Autodesk Fusion 360 part; units mm, degrees
(part 3 of 6)
  spline S740 degree 3 poles (-68.6412, -18.0684) (-68.8412, -19.3768) (-68.5019, -20.6874) (-67.7379, -21.7563) knots 0 0 0 0 1 1 1 1
  spline S741 degree 3 poles (-67.7379, -21.7563) (-67.4869, -22.0922) (-67.1872, -22.3895) (-66.7921, -22.5521) knots 0 0 0 0 1 1 1 1
  spline S742 degree 3 poles (-66.7921, -22.5521) (-66.7066, -22.5523) (-66.7066, -22.5523) (-66.6238, -22.5405) knots 0 0 0 0 1 1 1 1
  spline S743 degree 3 poles (-66.6238, -22.5405) (-66.5712, -22.5389) (-66.5187, -22.5373) (-66.4646, -22.5356) knots 0 0 0 0 1 1 1 1
  spline S744 degree 3 poles (-66.4646, -22.5356) (-66.4043, -22.5997) (-66.4043, -22.5997) (-66.3562, -22.6818) knots 0 0 0 0 1 1 1 1
  spline S745 degree 3 poles (-66.3562, -22.6818) (-66.0629, -23.057) (-65.7293, -23.2124) (-65.2682, -23.3032) knots 0 0 0 0 1 1 1 1
  spline S746 degree 3 poles (-65.2682, -23.3032) (-64.8355, -23.3775) (-64.8355, -23.3775) (-64.5079, -23.6467) knots 0 0 0 0 1 1 1 1
  spline S747 degree 3 poles (-64.5079, -23.6467) (-64.3934, -23.7401) (-64.3934, -23.7401) (-64.303, -23.7316) knots 0 0 0 0 1 1 1 1
  spline S748 degree 3 poles (-64.303, -23.7316) (-64.2502, -23.719) (-64.2502, -23.719) (-64.1964, -23.706) knots 0 0 0 0 1 1 1 1
  spline S749 degree 3 poles (-64.1964, -23.706) (-63.9469, -23.6555) (-63.7172, -23.6642) (-63.4643, -23.6796) knots 0 0 0 0 1 1 1 1
  spline S750 degree 3 poles (-63.4643, -23.6796) (-62.4889, -23.724) (-62.4889, -23.724) (-62.1287, -23.4647) knots 0 0 0 0 1 1 1 1
  spline S751 degree 3 poles (-62.1287, -23.4647) (-62.0488, -23.3538) (-61.9871, -23.2352) (-61.9247, -23.1138) knots 0 0 0 0 1 1 1 1
  spline S752 degree 3 poles (-61.9247, -23.1138) (-61.8889, -23.0471) (-61.8532, -22.9804) (-61.8173, -22.9138) knots 0 0 0 0 1 1 1 1
  spline S753 degree 3 poles (-61.8173, -22.9138) (-61.7921, -22.8662) (-61.7921, -22.8662) (-61.7664, -22.8176) knots 0 0 0 0 1 1 1 1
  spline S754 degree 3 poles (-61.7664, -22.8176) (-61.5666, -22.4407) (-61.3314, -22.1103) (-60.9949, -21.8423) knots 0 0 0 0 1 1 1 1
  spline S755 degree 3 poles (-60.9949, -21.8423) (-60.8309, -21.6988) (-60.7879, -21.5385) (-60.7711, -21.3252) knots 0 0 0 0 1 1 1 1
  spline S756 degree 3 poles (-60.7711, -21.3252) (-60.7791, -21.0767) (-60.8479, -20.9431) (-60.9972, -20.7455) knots 0 0 0 0 1 1 1 1
  spline S757 degree 3 poles (-60.9972, -20.7455) (-61.0269, -20.5521) (-60.9721, -20.3858) (-60.9221, -20.2004) knots 0 0 0 0 1 1 1 1
  spline S758 degree 3 poles (-60.9221, -20.2004) (-60.8997, -20.0941) (-60.9058, -20.0126) (-60.9382, -19.9089) knots 0 0 0 0 1 1 1 1
  spline S759 degree 3 poles (-60.9382, -19.9089) (-60.9049, -19.8925) (-60.8717, -19.8761) (-60.8374, -19.8592) knots 0 0 0 0 1 1 1 1
  spline S760 degree 3 poles (-60.8374, -19.8592) (-60.5508, -19.6929) (-60.3089, -19.433) (-60.2049, -19.1155) knots 0 0 0 0 1 1 1 1
  spline S761 degree 3 poles (-60.2049, -19.1155) (-60.1104, -18.7393) (-60.169, -18.4062) (-60.3535, -18.0709) knots 0 0 0 0 1 1 1 1
  spline S762 degree 3 poles (-60.3535, -18.0709) (-60.3718, -17.8493) (-60.3514, -17.638) (-60.3266, -17.4182) knots 0 0 0 0 1 1 1 1
  spline S763 degree 3 poles (-60.3266, -17.4182) (-60.2811, -16.9783) (-60.2704, -16.5662) (-60.3651, -16.1315) knots 0 0 0 0 1 1 1 1
  spline S764 degree 3 poles (-60.3651, -16.1315) (-60.3404, -16.1338) (-60.3158, -16.1361) (-60.2904, -16.1385) knots 0 0 0 0 1 1 1 1
  spline S765 degree 3 poles (-60.2904, -16.1385) (-60.0658, -16.1502) (-59.8801, -16.0893) (-59.6783, -16.0001) knots 0 0 0 0 1 1 1 1
  spline S766 degree 3 poles (-59.6783, -16.0001) (-59.3356, -15.8722) (-59.0125, -15.9703) (-58.6693, -16.0524) knots 0 0 0 0 1 1 1 1
  spline S767 degree 3 poles (-58.6693, -16.0524) (-56.6827, -16.5272) (-54.5948, -16.1567) (-52.6142, -15.7994) knots 0 0 0 0 1 1 1 1
  spline S768 degree 3 poles (-52.6142, -15.7994) (-52.425, -15.7652) (-52.2358, -15.7315) (-52.0466, -15.6978) knots 0 0 0 0 1 1 1 1
  spline S769 degree 3 poles (-52.0466, -15.6978) (-51.5093, -15.6021) (-50.9721, -15.5059) (-50.4349, -15.4093) knots 0 0 0 0 1 1 1 1
  spline S770 degree 3 poles (-50.4349, -15.4093) (-50.1364, -15.3556) (-49.8377, -15.3022) (-49.539, -15.2492) knots 0 0 0 0 1 1 1 1
  spline S771 degree 3 poles (-49.539, -15.2492) (-49.3825, -15.2214) (-49.2259, -15.1934) (-49.0695, -15.165) knots 0 0 0 0 1 1 1 1
  spline S772 degree 3 poles (-49.0695, -15.165) (-47.9373, -14.9598) (-46.7937, -14.7812) (-45.6425, -14.736) knots 0 0 0 0 1 1 1 1
  spline S773 degree 3 poles (-45.6425, -14.736) (-45.5861, -14.7334) (-45.5298, -14.7307) (-45.4735, -14.7279) knots 0 0 0 0 1 1 1 1
  spline S774 degree 3 poles (-45.4735, -14.7279) (-45.2474, -14.7174) (-45.0218, -14.7091) (-44.7954, -14.708) knots 0 0 0 0 1 1 1 1
  spline S775 degree 3 poles (-44.7954, -14.708) (-44.7994, -14.7532) (-44.8034, -14.7983) (-44.8075, -14.8449) knots 0 0 0 0 1 1 1 1
  spline S776 degree 3 poles (-44.8075, -14.8449) (-44.8816, -15.7919) (-44.8816, -15.7919) (-44.6213, -16.1643) knots 0 0 0 0 1 1 1 1
  spline S777 degree 3 poles (-44.6213, -16.1643) (-44.5265, -16.2347) (-44.4252, -16.2864) (-44.3195, -16.3383) knots 0 0 0 0 1 1 1 1
  spline S778 degree 3 poles (-44.3195, -16.3383) (-44.2905, -16.353) (-44.2615, -16.3677) (-44.2317, -16.3828) knots 0 0 0 0 1 1 1 1
  spline S779 degree 3 poles (-44.2317, -16.3828) (-44.1742, -16.4117) (-44.1167, -16.4403) (-44.0589, -16.4685) knots 0 0 0 0 1 1 1 1
  spline S780 degree 3 poles (-44.0589, -16.4685) (-43.9984, -16.4984) (-43.9388, -16.53) (-43.8796, -16.5622) knots 0 0 0 0 1 1 1 1
  spline S781 degree 3 poles (-43.8796, -16.5622) (-43.2204, -16.8977) (-42.2928, -16.9139) (-41.572, -16.8246) knots 0 0 0 0 1 1 1 1
  spline S782 degree 3 poles (-41.572, -16.8246) (-41.5398, -16.823) (-41.5077, -16.8213) (-41.4745, -16.8197) knots 0 0 0 0 1 1 1 1
  spline S783 degree 3 poles (-41.4745, -16.8197) (-41.3362, -16.8073) (-41.2458, -16.7972) (-41.1479, -16.694) knots 0 0 0 0 1 1 1 1
  spline S784 degree 3 poles (-41.1479, -16.694) (-40.9639, -16.4028) (-40.9726, -16.1477) (-41.0367, -15.8177) knots 0 0 0 0 1 1 1 1
  spline S785 degree 3 poles (-41.0367, -15.8177) (-41.094, -15.6049) (-41.2091, -15.4396) (-41.3857, -15.3047) knots 0 0 0 0 1 1 1 1
  spline S786 degree 3 poles (-41.3857, -15.3047) (-41.4121, -15.3093) (-41.4385, -15.314) (-41.4658, -15.3188) knots 0 0 0 0 1 1 1 1
  spline S787 degree 3 poles (-41.4658, -15.3188) (-41.4806, -15.2976) (-41.4954, -15.2763) (-41.5107, -15.2544) knots 0 0 0 0 1 1 1 1
  spline S788 degree 3 poles (-41.5107, -15.2544) (-41.5751, -15.1714) (-41.6453, -15.1045) (-41.7226, -15.0336) knots 0 0 0 0 1 1 1 1
  spline S789 degree 3 poles (-41.7226, -15.0336) (-41.6474, -15.0014) (-41.5722, -14.9692) (-41.497, -14.937) knots 0 0 0 0 1 1 1 1
  spline S790 degree 3 poles (-41.497, -14.937) (-41.4514, -14.9175) (-41.4058, -14.8979) (-41.3588, -14.8777) knots 0 0 0 0 1 1 1 1
  spline S791 degree 3 poles (-41.3588, -14.8777) (-41.2453, -14.8308) (-41.1322, -14.7907) (-41.0159, -14.7515) knots 0 0 0 0 1 1 1 1
  spline S792 degree 3 poles (-41.0159, -14.7515) (-40.6691, -14.6161) (-40.4632, -14.2783) (-40.3015, -13.9569) knots 0 0 0 0 1 1 1 1
  spline S793 degree 3 poles (-40.3015, -13.9569) (-40.2178, -13.7291) (-40.1926, -13.5214) (-40.2142, -13.2806) knots 0 0 0 0 1 1 1 1
  spline S794 degree 3 poles (-40.2142, -13.2806) (-40.105, -13.2803) (-40.0232, -13.2817) (-39.9196, -13.3113) knots 0 0 0 0 1 1 1 1
  spline S795 degree 3 poles (-39.9196, -13.3113) (-39.828, -13.4095) (-39.828, -13.4095) (-39.7728, -13.4871) knots 0 0 0 0 1 1 1 1
  spline S796 degree 3 poles (-39.7728, -13.4871) (-39.1827, -14.2043) (-38.1238, -14.3933) (-37.2636, -14.5675) knots 0 0 0 0 1 1 1 1
  spline S797 degree 3 poles (-37.2636, -14.5675) (-37.1583, -14.5891) (-37.053, -14.6108) (-36.9477, -14.6327) knots 0 0 0 0 1 1 1 1
  spline S798 degree 3 poles (-36.9477, -14.6327) (-36.8831, -14.6461) (-36.8183, -14.6593) (-36.7536, -14.6724) knots 0 0 0 0 1 1 1 1
  spline S799 degree 3 poles (-36.7536, -14.6724) (-36.5691, -14.7103) (-36.3908, -14.7577) (-36.2115, -14.8155) knots 0 0 0 0 1 1 1 1
  spline S800 degree 3 poles (-36.2115, -14.8155) (-36.14, -14.8341) (-36.14, -14.8341) (-36.0599, -14.82) knots 0 0 0 0 1 1 1 1
  spline S801 degree 3 poles (-36.0599, -14.82) (-36.0685, -14.8488) (-36.077, -14.8775) (-36.0858, -14.9072) knots 0 0 0 0 1 1 1 1
  spline S802 degree 3 poles (-36.0858, -14.9072) (-36.1556, -14.9418) (-36.1556, -14.9418) (-36.244, -14.9684) knots 0 0 0 0 1 1 1 1
  spline S803 degree 3 poles (-36.244, -14.9684) (-36.2782, -14.9796) (-36.3123, -14.9909) (-36.3475, -15.0025) knots 0 0 0 0 1 1 1 1
  spline S804 degree 3 poles (-36.3475, -15.0025) (-36.385, -15.0145) (-36.4225, -15.0265) (-36.4612, -15.0389) knots 0 0 0 0 1 1 1 1
  spline S805 degree 3 poles (-36.4612, -15.0389) (-36.4999, -15.0515) (-36.5387, -15.0642) (-36.5786, -15.0773) knots 0 0 0 0 1 1 1 1
  spline S806 degree 3 poles (-36.5786, -15.0773) (-36.6619, -15.1045) (-36.7452, -15.1316) (-36.8286, -15.1585) knots 0 0 0 0 1 1 1 1
  spline S807 degree 3 poles (-36.8286, -15.1585) (-36.958, -15.2003) (-37.0873, -15.2425) (-37.2165, -15.2849) knots 0 0 0 0 1 1 1 1
  spline S808 degree 3 poles (-37.2165, -15.2849) (-37.5564, -15.3961) (-37.8965, -15.5064) (-38.2368, -15.6164) knots 0 0 0 0 1 1 1 1
  spline S809 degree 3 poles (-38.2368, -15.6164) (-38.3584, -15.6559) (-38.4799, -15.6957) (-38.6015, -15.7354) knots 0 0 0 0 1 1 1 1
  spline S810 degree 3 poles (-38.6015, -15.7354) (-38.6442, -15.749) (-38.6869, -15.7626) (-38.7309, -15.7766) knots 0 0 0 0 1 1 1 1
  spline S811 degree 3 poles (-38.7309, -15.7766) (-38.7688, -15.789) (-38.8066, -15.8014) (-38.8456, -15.8141) knots 0 0 0 0 1 1 1 1
  spline S812 degree 3 poles (-38.8456, -15.8141) (-38.8777, -15.8244) (-38.9098, -15.8347) (-38.9428, -15.8454) knots 0 0 0 0 1 1 1 1
  spline S813 degree 3 poles (-38.9428, -15.8454) (-38.9659, -15.856) (-38.989, -15.8667) (-39.0127, -15.8776) knots 0 0 0 0 1 1 1 1
  spline S814 degree 3 poles (-39.0127, -15.8776) (-39.064, -16.0501) (-39.0117, -16.2422) (-38.9897, -16.4183) knots 0 0 0 0 1 1 1 1
  spline S815 degree 3 poles (-38.9897, -16.4183) (-38.9829, -16.4809) (-38.9829, -16.4809) (-38.976, -16.5447) knots 0 0 0 0 1 1 1 1
  spline S816 degree 3 poles (-38.976, -16.5447) (-38.9451, -16.7912) (-38.9094, -16.9616) (-38.7466, -17.1525) knots 0 0 0 0 1 1 1 1
  spline S817 degree 3 poles (-38.7466, -17.1525) (-38.5182, -17.2701) (-38.3218, -17.2898) (-38.0703, -17.2398) knots 0 0 0 0 1 1 1 1
  spline S818 degree 3 poles (-38.0703, -17.2398) (-37.993, -17.2137) (-37.9161, -17.1863) (-37.8395, -17.1578) knots 0 0 0 0 1 1 1 1
  spline S819 degree 3 poles (-37.8395, -17.1578) (-37.0677, -16.8843) (-36.2352, -16.9908) (-35.4358, -17.0521) knots 0 0 0 0 1 1 1 1
  spline S820 degree 3 poles (-35.4358, -17.0521) (-34.7031, -17.1078) (-34.0053, -17.132) (-33.2842, -16.9742) knots 0 0 0 0 1 1 1 1
  spline S821 degree 3 poles (-33.2842, -16.9742) (-33.276, -17.0018) (-33.2678, -17.0295) (-33.2593, -17.0579) knots 0 0 0 0 1 1 1 1
  spline S822 degree 3 poles (-33.2593, -17.0579) (-33.0671, -17.4752) (-32.5518, -17.7504) (-32.1451, -17.9145) knots 0 0 0 0 1 1 1 1
  spline S823 degree 3 poles (-32.1451, -17.9145) (-31.6456, -18.089) (-31.1293, -18.1169) (-30.6051, -18.1128) knots 0 0 0 0 1 1 1 1
  spline S824 degree 3 poles (-30.6051, -18.1128) (-30.5551, -18.1131) (-30.5052, -18.1134) (-30.4537, -18.1137) knots 0 0 0 0 1 1 1 1
  spline S825 degree 3 poles (-30.4537, -18.1137) (-30.2637, -18.0993) (-30.1747, -18.031) (-30.0183, -17.9267) knots 0 0 0 0 1 1 1 1
  spline S826 degree 3 poles (-30.0183, -17.9267) (-29.9953, -17.9746) (-29.9724, -18.0225) (-29.9488, -18.0719) knots 0 0 0 0 1 1 1 1
  spline S827 degree 3 poles (-29.9488, -18.0719) (-29.6863, -18.5524) (-29.2614, -18.9058) (-28.739, -19.0617) knots 0 0 0 0 1 1 1 1
  spline S828 degree 3 poles (-28.739, -19.0617) (-28.3779, -19.1626) (-28.0211, -19.2161) (-27.668, -19.0613) knots 0 0 0 0 1 1 1 1
  spline S829 degree 3 poles (-27.668, -19.0613) (-27.5114, -18.9684) (-27.4277, -18.8659) (-27.3626, -18.6976) knots 0 0 0 0 1 1 1 1
  spline S830 degree 3 poles (-27.3626, -18.6976) (-27.3559, -18.5596) (-27.3559, -18.5596) (-27.3649, -18.4502) knots 0 0 0 0 1 1 1 1
  spline S831 degree 3 poles (-27.3649, -18.4502) (-27.1789, -18.5763) (-27.0065, -18.7141) (-26.8336, -18.8574) knots 0 0 0 0 1 1 1 1
  spline S832 degree 3 poles (-26.8336, -18.8574) (-25.8457, -19.6635) (-24.4693, -20.4549) (-23.14, -20.3902) knots 0 0 0 0 1 1 1 1
  spline S833 degree 3 poles (-23.14, -20.3902) (-22.9866, -20.3473) (-22.9116, -20.291) (-22.8156, -20.1652) knots 0 0 0 0 1 1 1 1
  spline S834 degree 3 poles (-22.8156, -20.1652) (-22.7953, -20.139) (-22.7749, -20.1128) (-22.754, -20.0857) knots 0 0 0 0 1 1 1 1
  spline S835 degree 3 poles (-22.754, -20.0857) (-22.739, -20.0657) (-22.7241, -20.0457) (-22.7087, -20.025) knots 0 0 0 0 1 1 1 1
  spline S836 degree 3 poles (-22.7087, -20.025) (-22.6443, -20.1421) (-22.5821, -20.2595) (-22.5234, -20.3796) knots 0 0 0 0 1 1 1 1
  spline S837 degree 3 poles (-22.5234, -20.3796) (-21.9291, -21.5595) (-20.6318, -22.2811) (-19.4264, -22.7095) knots 0 0 0 0 1 1 1 1
  spline S838 degree 3 poles (-19.4264, -22.7095) (-18.9788, -22.8304) (-18.5829, -22.8182) (-18.1633, -22.6107) knots 0 0 0 0 1 1 1 1
  spline S839 degree 3 poles (-18.1633, -22.6107) (-18.0483, -22.5271) (-17.9669, -22.4305) (-17.8852, -22.3138) knots 0 0 0 0 1 1 1 1
  spline S840 degree 3 poles (-17.8852, -22.3138) (-17.8567, -22.0715) (-17.9152, -21.8824) (-18.0605, -21.6893) knots 0 0 0 0 1 1 1 1
  spline S841 degree 3 poles (-18.0605, -21.6893) (-18.2688, -21.4713) (-18.5357, -21.3675) (-18.8195, -21.2824) knots 0 0 0 0 1 1 1 1
  spline S842 degree 3 poles (-18.8195, -21.2824) (-18.9043, -21.2593) (-18.9043, -21.2593) (-18.9526, -21.1802) knots 0 0 0 0 1 1 1 1
  spline S843 degree 3 poles (-18.9526, -21.1802) (-18.9261, -21.1665) (-18.8997, -21.1529) (-18.8724, -21.1388) knots 0 0 0 0 1 1 1 1
  spline S844 degree 3 poles (-18.8724, -21.1388) (-18.7401, -21.0464) (-18.6537, -20.9322) (-18.5594, -20.8037) knots 0 0 0 0 1 1 1 1
  spline S845 degree 3 poles (-18.5594, -20.8037) (-18.5331, -20.7686) (-18.5331, -20.7686) (-18.5062, -20.7329) knots 0 0 0 0 1 1 1 1
  spline S846 degree 3 poles (-18.5062, -20.7329) (-18.4236, -20.6226) (-18.3424, -20.5115) (-18.2644, -20.3979) knots 0 0 0 0 1 1 1 1
  spline S847 degree 3 poles (-18.2644, -20.3979) (-18.2324, -20.4233) (-18.2004, -20.4486) (-18.1674, -20.4748) knots 0 0 0 0 1 1 1 1
  spline S848 degree 3 poles (-18.1674, -20.4748) (-17.7298, -20.8181) (-17.2734, -21.1066) (-16.7784, -21.3598) knots 0 0 0 0 1 1 1 1
  spline S849 degree 3 poles (-16.7784, -21.3598) (-16.5763, -21.4634) (-16.3766, -21.5705) (-16.179, -21.6825) knots 0 0 0 0 1 1 1 1
  spline S850 degree 3 poles (-16.179, -21.6825) (-16.1408, -21.7041) (-16.1026, -21.7256) (-16.0633, -21.7478) knots 0 0 0 0 1 1 1 1
  spline S851 degree 3 poles (-16.0633, -21.7478) (-15.8503, -21.8737) (-15.6798, -22.003) (-15.5076, -22.1812) knots 0 0 0 0 1 1 1 1
  spline S852 degree 3 poles (-15.5076, -22.1812) (-15.1305, -22.5482) (-14.4719, -22.7942) (-13.9467, -22.7924) knots 0 0 0 0 1 1 1 1
  spline S853 degree 3 poles (-13.9467, -22.7924) (-13.7622, -22.7691) (-13.6383, -22.6968) (-13.5022, -22.5737) knots 0 0 0 0 1 1 1 1
  spline S854 degree 3 poles (-13.5022, -22.5737) (-13.4682, -22.5272) (-13.4352, -22.4801) (-13.4032, -22.4323) knots 0 0 0 0 1 1 1 1
  spline S855 degree 3 poles (-13.4032, -22.4323) (-13.3735, -22.4075) (-13.3438, -22.3826) (-13.3132, -22.357) knots 0 0 0 0 1 1 1 1
  spline S856 degree 3 poles (-13.3132, -22.357) (-13.1964, -22.2519) (-13.14, -22.1775) (-13.1248, -22.0182) knots 0 0 0 0 1 1 1 1
  spline S857 degree 3 poles (-13.1248, -22.0182) (-13.1272, -21.6444) (-13.2828, -21.3286) (-13.5456, -21.0684) knots 0 0 0 0 1 1 1 1
  spline S858 degree 3 poles (-13.5456, -21.0684) (-13.7172, -20.9144) (-13.8973, -20.7722) (-14.0803, -20.632) knots 0 0 0 0 1 1 1 1
  spline S859 degree 3 poles (-14.0803, -20.632) (-14.5227, -20.289) (-14.9136, -19.9414) (-15.1701, -19.4393) knots 0 0 0 0 1 1 1 1
  spline S860 degree 3 poles (-15.1701, -19.4393) (-15.0261, -19.4638) (-14.8823, -19.4895) (-14.7385, -19.5155) knots 0 0 0 0 1 1 1 1
  spline S861 degree 3 poles (-14.7385, -19.5155) (-14.698, -19.5224) (-14.6574, -19.5293) (-14.6157, -19.5364) knots 0 0 0 0 1 1 1 1
  spline S862 degree 3 poles (-14.6157, -19.5364) (-14.3073, -19.5929) (-14.0901, -19.6827) (-13.8472, -19.885) knots 0 0 0 0 1 1 1 1
  spline S863 degree 3 poles (-13.8472, -19.885) (-13.8189, -19.9083) (-13.7906, -19.9316) (-13.7615, -19.9556) knots 0 0 0 0 1 1 1 1
  spline S864 degree 3 poles (-13.7615, -19.9556) (-13.7279, -19.9836) (-13.6943, -20.0116) (-13.6597, -20.0404) knots 0 0 0 0 1 1 1 1
  spline S865 degree 3 poles (-13.6597, -20.0404) (-11.7063, -21.6601) (-11.7063, -21.6601) (-10.6489, -21.5847) knots 0 0 0 0 1 1 1 1
  spline S866 degree 3 poles (-10.6489, -21.5847) (-10.4516, -21.556) (-10.2712, -21.5209) (-10.1149, -21.3918) knots 0 0 0 0 1 1 1 1
  spline S867 degree 3 poles (-10.1149, -21.3918) (-9.8826, -21.0789) (-9.7948, -20.6136) (-9.8257, -20.2318) knots 0 0 0 0 1 1 1 1
  spline S868 degree 3 poles (-9.8257, -20.2318) (-9.8623, -20.2138) (-9.8988, -20.1958) (-9.9365, -20.1773) knots 0 0 0 0 1 1 1 1
  spline S869 degree 3 poles (-9.9365, -20.1773) (-9.9854, -20.1529) (-10.0343, -20.1286) (-10.0831, -20.1042) knots 0 0 0 0 1 1 1 1
  spline S870 degree 3 poles (-10.0831, -20.1042) (-10.1309, -20.0805) (-10.1787, -20.0569) (-10.2279, -20.0325) knots 0 0 0 0 1 1 1 1
  spline S871 degree 3 poles (-10.2279, -20.0325) (-10.3628, -19.9599) (-10.4832, -19.8828) (-10.6056, -19.791) knots 0 0 0 0 1 1 1 1
  spline S872 degree 3 poles (-10.6056, -19.791) (-10.6402, -19.7654) (-10.6747, -19.7398) (-10.7103, -19.7135) knots 0 0 0 0 1 1 1 1
  spline S873 degree 3 poles (-10.7103, -19.7135) (-10.8239, -19.5954) (-10.8735, -19.4701) (-10.9265, -19.3184) knots 0 0 0 0 1 1 1 1
  spline S874 degree 3 poles (-10.9265, -19.3184) (-10.9414, -19.278) (-10.9414, -19.278) (-10.9565, -19.2369) knots 0 0 0 0 1 1 1 1
  spline S875 degree 3 poles (-10.9565, -19.2369) (-10.9806, -19.1712) (-11.0041, -19.1053) (-11.0274, -19.0392) knots 0 0 0 0 1 1 1 1
  spline S876 degree 3 poles (-11.0274, -19.0392) (-10.9636, -19.0144) (-10.8998, -18.9895) (-10.8341, -18.9639) knots 0 0 0 0 1 1 1 1
  spline S877 degree 3 poles (-10.8341, -18.9639) (-10.8183, -18.9908) (-10.8025, -19.0178) (-10.7863, -19.0456) knots 0 0 0 0 1 1 1 1
  spline S878 degree 3 poles (-10.7863, -19.0456) (-10.7181, -19.1508) (-10.6447, -19.2389) (-10.5605, -19.3316) knots 0 0 0 0 1 1 1 1
  spline S879 degree 3 poles (-10.5605, -19.3316) (-10.5292, -19.3662) (-10.498, -19.4007) (-10.4657, -19.4363) knots 0 0 0 0 1 1 1 1
  spline S880 degree 3 poles (-10.4657, -19.4363) (-10.4324, -19.4729) (-10.399, -19.5095) (-10.3647, -19.5472) knots 0 0 0 0 1 1 1 1
  spline S881 degree 3 poles (-10.3647, -19.5472) (-10.3304, -19.5849) (-10.2961, -19.6227) (-10.2608, -19.6616) knots 0 0 0 0 1 1 1 1
  spline S882 degree 3 poles (-10.2608, -19.6616) (-10.1906, -19.739) (-10.1203, -19.8164) (-10.05, -19.8936) knots 0 0 0 0 1 1 1 1
  spline S883 degree 3 poles (-10.05, -19.8936) (-9.9562, -19.9968) (-9.8627, -20.1001) (-9.7694, -20.2036) knots 0 0 0 0 1 1 1 1
  spline S884 degree 3 poles (-9.7694, -20.2036) (-9.7156, -20.2631) (-9.6619, -20.3225) (-9.6082, -20.3819) knots 0 0 0 0 1 1 1 1
  spline S885 degree 3 poles (-9.6082, -20.3819) (-9.584, -20.4088) (-9.5598, -20.4356) (-9.5348, -20.4633) knots 0 0 0 0 1 1 1 1
  spline S886 degree 3 poles (-9.5348, -20.4633) (-9.4895, -20.5133) (-9.4437, -20.5628) (-9.3975, -20.6119) knots 0 0 0 0 1 1 1 1
  spline S887 degree 3 poles (-9.3975, -20.6119) (-9.3323, -20.6811) (-9.3323, -20.6811) (-9.275, -20.7566) knots 0 0 0 0 1 1 1 1
  spline S888 degree 3 poles (-9.275, -20.7566) (-9.1872, -20.861) (-9.1313, -20.9227) (-8.9917, -20.9354) knots 0 0 0 0 1 1 1 1
  spline S889 degree 3 poles (-8.9917, -20.9354) (-8.8845, -20.925) (-8.7835, -20.9055) (-8.6785, -20.8815) knots 0 0 0 0 1 1 1 1
  spline S890 degree 3 poles (-8.6785, -20.8815) (-8.6429, -20.8749) (-8.6073, -20.8684) (-8.5706, -20.8617) knots 0 0 0 0 1 1 1 1
  spline S891 degree 3 poles (-8.5706, -20.8617) (-8.3384, -20.8146) (-8.207, -20.7524) (-8.0515, -20.5696) knots 0 0 0 0 1 1 1 1
  spline S892 degree 3 poles (-8.0515, -20.5696) (-7.9886, -20.4625) (-7.9808, -20.3722) (-7.9672, -20.2488) knots 0 0 0 0 1 1 1 1
  spline S893 degree 3 poles (-7.9672, -20.2488) (-7.9588, -20.1749) (-7.9588, -20.1749) (-7.9502, -20.0996) knots 0 0 0 0 1 1 1 1
  spline S894 degree 3 poles (-7.9502, -20.0996) (-7.9445, -20.0455) (-7.9387, -19.9913) (-7.933, -19.9371) knots 0 0 0 0 1 1 1 1
  spline S895 degree 3 poles (-7.933, -19.9371) (-7.9267, -19.8805) (-7.9204, -19.8238) (-7.914, -19.7672) knots 0 0 0 0 1 1 1 1
  spline S896 degree 3 poles (-7.914, -19.7672) (-7.8939, -19.586) (-7.8747, -19.4048) (-7.8555, -19.2235) knots 0 0 0 0 1 1 1 1
  spline S897 degree 3 poles (-7.8555, -19.2235) (-7.8524, -19.1939) (-7.8492, -19.1643) (-7.846, -19.1338) knots 0 0 0 0 1 1 1 1
  spline S898 degree 3 poles (-7.846, -19.1338) (-7.7919, -18.6232) (-7.7389, -18.1125) (-7.6871, -17.6016) knots 0 0 0 0 1 1 1 1
  spline S899 degree 3 poles (-7.6871, -17.6016) (-7.6717, -17.4496) (-7.656, -17.2976) (-7.6401, -17.1455) knots 0 0 0 0 1 1 1 1
  spline S900 degree 3 poles (-7.6401, -17.1455) (-7.6343, -17.0889) (-7.6285, -17.0323) (-7.6229, -16.9756) knots 0 0 0 0 1 1 1 1
  spline S901 degree 3 poles (-7.6229, -16.9756) (-7.5229, -15.9721) (-7.1763, -15.2785) (-6.5968, -14.4733) knots 0 0 0 0 1 1 1 1
  spline S902 degree 3 poles (-6.5968, -14.4733) (-6.094, -13.7574) (-5.8647, -13.0472) (-5.8847, -12.1718) knots 0 0 0 0 1 1 1 1
  spline S903 degree 3 poles (-5.8847, -12.1718) (-5.9176, -10.6288) (-5.5589, -9.1781) (-5.1585, -7.7002) knots 0 0 0 0 1 1 1 1
  spline S904 degree 3 poles (-5.1585, -7.7002) (-4.8304, -6.4848) (-4.5331, -5.2756) (-4.5072, -4.0104) knots 0 0 0 0 1 1 1 1
  spline S905 degree 3 poles (-4.5072, -4.0104) (-4.5058, -3.977) (-4.5044, -3.9435) (-4.503, -3.9091) knots 0 0 0 0 1 1 1 1
  spline S906 degree 3 poles (-4.503, -3.9091) (-4.5031, -3.653) (-4.5935, -3.5218) (-4.7651, -3.3382) knots 0 0 0 0 1 1 1 1
  spline S907 degree 3 poles (-4.7651, -3.3382) (-4.7886, -3.3119) (-4.8122, -3.2856) (-4.8364, -3.2585) knots 0 0 0 0 1 1 1 1
  spline S908 degree 3 poles (-4.8364, -3.2585) (-5.0381, -3.0374) (-5.2552, -2.8411) (-5.4896, -2.6553) knots 0 0 0 0 1 1 1 1
  spline S909 degree 3 poles (-5.4896, -2.6553) (-5.5229, -2.627) (-5.5561, -2.5987) (-5.5903, -2.5696) knots 0 0 0 0 1 1 1 1
  spline S910 degree 3 poles (-5.5903, -2.5696) (-5.8874, -2.323) (-6.2137, -2.1449) (-6.5594, -1.9764) knots 0 0 0 0 1 1 1 1
  spline S911 degree 3 poles (-6.5594, -1.9764) (-6.5958, -1.9584) (-6.6322, -1.9404) (-6.6697, -1.9218) knots 0 0 0 0 1 1 1 1
  spline S912 degree 3 poles (-6.6697, -1.9218) (-6.8187, -1.8813) (-6.9456, -1.902) (-7.094, -1.9313) knots 0 0 0 0 1 1 1 1
  spline S913 degree 3 poles (-7.094, -1.9313) (-7.1224, -1.9367) (-7.1508, -1.9422) (-7.18, -1.9478) knots 0 0 0 0 1 1 1 1
  spline S914 degree 3 poles (-7.18, -1.9478) (-7.4344, -2.0006) (-7.6602, -2.0563) (-7.8229, -2.2689) knots 0 0 0 0 1 1 1 1
  spline S915 degree 3 poles (-7.8229, -2.2689) (-7.8889, -2.3762) (-7.9422, -2.4775) (-7.9781, -2.5984) knots 0 0 0 0 1 1 1 1
  spline S916 degree 3 poles (-7.9781, -2.5984) (-7.9882, -2.5642) (-7.9982, -2.5301) (-8.0086, -2.495) knots 0 0 0 0 1 1 1 1
  spline S917 degree 3 poles (-8.0086, -2.495) (-8.1573, -2.0202) (-8.1573, -2.0202) (-8.3527, -1.8796) knots 0 0 0 0 1 1 1 1
  spline S918 degree 3 poles (-8.3527, -1.8796) (-8.6228, -1.7428) (-8.8578, -1.7785) (-9.1421, -1.8535) knots 0 0 0 0 1 1 1 1
  spline S919 degree 3 poles (-9.1421, -1.8535) (-9.1839, -1.8643) (-9.2257, -1.8751) (-9.2688, -1.8862) knots 0 0 0 0 1 1 1 1
  spline S920 degree 3 poles (-9.2688, -1.8862) (-9.7663, -2.0335) (-10.1303, -2.3461) (-10.3832, -2.7964) knots 0 0 0 0 1 1 1 1
  spline S921 degree 3 poles (-10.3832, -2.7964) (-10.5393, -3.1129) (-10.6428, -3.438) (-10.7447, -3.7755) knots 0 0 0 0 1 1 1 1
  spline S922 degree 3 poles (-10.7447, -3.7755) (-10.9034, -4.3429) (-10.9034, -4.3429) (-11.2681, -4.7894) knots 0 0 0 0 1 1 1 1
  spline S923 degree 3 poles (-11.2681, -4.7894) (-11.2627, -4.8975) (-11.2572, -5.0056) (-11.2516, -5.117) knots 0 0 0 0 1 1 1 1
  spline S924 degree 3 poles (-11.2516, -5.117) (-14.8872, -5.758) (-18.5228, -6.3991) (-22.2686, -7.0596) knots 0 0 0 0 1 1 1 1
  spline S925 degree 3 poles (-22.2686, -7.0596) (-22.1952, -6.6835) (-22.1271, -6.3847) (-21.9805, -6.0432) knots 0 0 0 0 1 1 1 1
  spline S926 degree 3 poles (-21.9805, -6.0432) (-21.947, -5.9622) (-21.9137, -5.8812) (-21.8806, -5.8) knots 0 0 0 0 1 1 1 1
  spline S927 degree 3 poles (-21.8806, -5.8) (-21.8646, -5.761) (-21.8486, -5.7219) (-21.8321, -5.6817) knots 0 0 0 0 1 1 1 1
  spline S928 degree 3 poles (-21.8321, -5.6817) (-21.771, -5.5287) (-21.7155, -5.3745) (-21.6639, -5.2181) knots 0 0 0 0 1 1 1 1
  spline S929 degree 3 poles (-21.6639, -5.2181) (-21.6549, -5.1919) (-21.6459, -5.1658) (-21.6367, -5.1389) knots 0 0 0 0 1 1 1 1
  spline S930 degree 3 poles (-21.6367, -5.1389) (-21.5949, -5.0103) (-21.5724, -4.8984) (-21.5656, -4.763) knots 0 0 0 0 1 1 1 1
  spline S931 degree 3 poles (-21.5656, -4.763) (-21.5569, -4.6005) (-21.5427, -4.5004) (-21.4646, -4.3568) knots 0 0 0 0 1 1 1 1
  spline S932 degree 3 poles (-21.4646, -4.3568) (-21.2232, -4.1628) (-20.9119, -4.0685) (-20.6256, -3.961) knots 0 0 0 0 1 1 1 1
  spline S933 degree 3 poles (-20.6256, -3.961) (-20.5479, -3.9297) (-20.4701, -3.8983) (-20.3925, -3.8668) knots 0 0 0 0 1 1 1 1
  spline S934 degree 3 poles (-20.3925, -3.8668) (-19.2941, -3.4304) (-18.1362, -3.0868) (-16.9847, -2.8233) knots 0 0 0 0 1 1 1 1
  spline S935 degree 3 poles (-16.9847, -2.8233) (-16.9514, -2.8157) (-16.9182, -2.8081) (-16.884, -2.8002) knots 0 0 0 0 1 1 1 1
  spline S936 degree 3 poles (-16.884, -2.8002) (-15.7502, -2.5409) (-14.6132, -2.3132) (-13.4663, -2.1197) knots 0 0 0 0 1 1 1 1
  spline S937 degree 3 poles (-13.4663, -2.1197) (-13.4231, -2.1124) (-13.3799, -2.1051) (-13.3354, -2.0975) knots 0 0 0 0 1 1 1 1
  spline S938 degree 3 poles (-13.3354, -2.0975) (-13.2551, -2.0839) (-13.1747, -2.0705) (-13.0942, -2.0573) knots 0 0 0 0 1 1 1 1
  spline S939 degree 3 poles (-13.0942, -2.0573) (-12.8951, -2.0237) (-12.71, -1.9796) (-12.519, -1.912) knots 0 0 0 0 1 1 1 1
  spline S940 degree 3 poles (-12.519, -1.912) (-12.1866, -1.8318) (-11.8696, -1.8008) (-11.5294, -1.7994) knots 0 0 0 0 1 1 1 1
  spline S941 degree 3 poles (-11.5294, -1.7994) (-11.2077, -1.7971) (-10.8995, -1.7628) (-10.5827, -1.7074) knots 0 0 0 0 1 1 1 1
  spline S942 degree 3 poles (-10.5827, -1.7074) (-10.5426, -1.7005) (-10.5025, -1.6937) (-10.4612, -1.6866) knots 0 0 0 0 1 1 1 1
  spline S943 degree 3 poles (-10.4612, -1.6866) (-10.2892, -1.6546) (-10.1469, -1.6216) (-9.9885, -1.545) knots 0 0 0 0 1 1 1 1
  spline S944 degree 3 poles (-9.9885, -1.545) (-9.4797, -1.3046) (-8.7207, -1.3939) (-8.1706, -1.375) knots 0 0 0 0 1 1 1 1
  spline S945 degree 3 poles (-8.1706, -1.375) (-8.1194, -1.3732) (-8.0681, -1.3713) (-8.0154, -1.3694) knots 0 0 0 0 1 1 1 1
  spline S946 degree 3 poles (-8.0154, -1.3694) (-7.2308, -1.3415) (-6.4478, -1.3301) (-5.6628, -1.3458) knots 0 0 0 0 1 1 1 1
  spline S947 degree 3 poles (-5.6628, -1.3458) (-5.3444, -1.3509) (-5.0427, -1.3467) (-4.7299, -1.2834) knots 0 0 0 0 1 1 1 1
  spline S948 degree 3 poles (-4.7299, -1.2834) (-3.9008, -1.1164) (-3.0464, -1.1732) (-2.2073, -1.2116) knots 0 0 0 0 1 1 1 1
  spline S949 degree 3 poles (-2.2073, -1.2116) (-0.9415, -1.2674) (-0.9415, -1.2674) (-0.4937, -1.2373) knots 0 0 0 0 1 1 1 1
  spline S950 degree 3 poles (-0.4937, -1.2373) (-0.4641, -1.2358) (-0.4346, -1.2343) (-0.4042, -1.2327) knots 0 0 0 0 1 1 1 1
  spline S951 degree 3 poles (-0.4042, -1.2327) (-0.2529, -1.2231) (-0.1135, -1.2029) (0.0271, -1.1455) knots 0 0 0 0 1 1 1 1
  spline S952 degree 3 poles (0.0271, -1.1455) (0.1572, -0.9806) (0.1982, -0.7652) (0.1812, -0.5579) knots 0 0 0 0 1 1 1 1
  spline S953 degree 3 poles (0.1812, -0.5579) (0.1362, -0.2594) (0.0544, -0.0507) (-0.1258, 0.1907) knots 0 0 0 0 1 1 1 1
  spline S954 degree 3 poles (-0.1258, 0.1907) (-0.1456, 0.2181) (-0.1655, 0.2455) (-0.1859, 0.2738) knots 0 0 0 0 1 1 1 1
  spline S955 degree 3 poles (-0.1859, 0.2738) (-0.304, 0.4287) (-0.4302, 0.5522) (-0.5806, 0.6759) knots 0 0 0 0 1 1 1 1
  spline S956 degree 3 poles (-0.5806, 0.6759) (-0.8356, 0.8941) (-0.9925, 1.164) (-1.1627, 1.45) knots 0 0 0 0 1 1 1 1
  spline S957 degree 3 poles (-1.1627, 1.45) (-1.4357, 1.9086) (-1.7257, 2.375) (-2.2417, 2.5852) knots 0 0 0 0 1 1 1 1
  spline S958 degree 3 poles (-2.2417, 2.5852) (-2.4109, 2.5947) (-2.5646, 2.5627) (-2.7298, 2.5275) knots 0 0 0 0 1 1 1 1
  spline S959 degree 3 poles (-2.7298, 2.5275) (-3.2147, 2.443) (-3.6642, 2.4353) (-4.1542, 2.4646) knots 0 0 0 0 1 1 1 1
  spline S960 degree 3 poles (-4.1542, 2.4646) (-4.3504, 2.476) (-4.5466, 2.4844) (-4.7429, 2.493) knots 0 0 0 0 1 1 1 1
  spline S961 degree 3 poles (-4.7429, 2.493) (-4.8409, 2.4973) (-4.9389, 2.5019) (-5.0369, 2.5067) knots 0 0 0 0 1 1 1 1
  spline S962 degree 3 poles (-5.0369, 2.5067) (-5.9674, 2.551) (-6.8135, 2.4127) (-7.5391, 1.8097) knots 0 0 0 0 1 1 1 1
  spline S963 degree 3 poles (-7.5391, 1.8097) (-8.0194, 1.433) (-8.6391, 1.3625) (-9.2229, 1.2631) knots 0 0 0 0 1 1 1 1
  spline S964 degree 3 poles (-9.2229, 1.2631) (-9.3505, 1.2413) (-9.4779, 1.2189) (-9.6054, 1.1965) knots 0 0 0 0 1 1 1 1
  spline S965 degree 3 poles (-9.6054, 1.1965) (-9.8566, 1.1526) (-10.1081, 1.111) (-10.36, 1.0711) knots 0 0 0 0 1 1 1 1
  spline S966 degree 3 poles (-10.36, 1.0711) (-10.4023, 1.0644) (-10.4446, 1.0577) (-10.4881, 1.0508) knots 0 0 0 0 1 1 1 1
  spline S967 degree 3 poles (-10.4881, 1.0508) (-10.6126, 1.0315) (-10.7372, 1.0132) (-10.8619, 0.9953) knots 0 0 0 0 1 1 1 1
  spline S968 degree 3 poles (-10.8619, 0.9953) (-10.9174, 0.9867) (-10.9174, 0.9867) (-10.974, 0.978) knots 0 0 0 0 1 1 1 1
  spline S969 degree 3 poles (-10.974, 0.978) (-11.2972, 0.9338) (-11.5784, 0.9851) (-11.8939, 1.055) knots 0 0 0 0 1 1 1 1
  spline S970 degree 3 poles (-11.8939, 1.055) (-12.2253, 1.1251) (-12.5627, 1.1284) (-12.9002, 1.1365) knots 0 0 0 0 1 1 1 1
  spline S971 degree 3 poles (-12.9002, 1.1365) (-13.0139, 1.1397) (-13.1274, 1.1451) (-13.2411, 1.1509) knots 0 0 0 0 1 1 1 1
  spline S972 degree 3 poles (-13.2411, 1.1509) (-13.7053, 1.1693) (-14.1136, 1.1145) (-14.5649, 1.0055) knots 0 0 0 0 1 1 1 1
  spline S973 degree 3 poles (-14.5649, 1.0055) (-15.1242, 0.8735) (-15.6961, 0.8743) (-16.2324, 1.1096) knots 0 0 0 0 1 1 1 1
  spline S974 degree 3 poles (-16.2324, 1.1096) (-16.3176, 1.1114) (-16.3176, 1.1114) (-16.415, 1.1038) knots 0 0 0 0 1 1 1 1
  spline S975 degree 3 poles (-16.415, 1.1038) (-16.47, 1.1002) (-16.47, 1.1002) (-16.526, 1.0964) knots 0 0 0 0 1 1 1 1
  spline S976 degree 3 poles (-16.526, 1.0964) (-16.5659, 1.0937) (-16.6058, 1.0909) (-16.6469, 1.0881) knots 0 0 0 0 1 1 1 1
  spline S977 degree 3 poles (-16.6469, 1.0881) (-17.7034, 1.0323) (-18.7383, 1.1918) (-19.7831, 1.3297) knots 0 0 0 0 1 1 1 1
  spline S978 degree 3 poles (-19.7831, 1.3297) (-20.4379, 1.4161) (-21.0924, 1.501) (-21.7523, 1.5355) knots 0 0 0 0 1 1 1 1
  spline S979 degree 3 poles (-21.7523, 1.5355) (-21.7869, 1.5374) (-21.8215, 1.5392) (-21.8571, 1.541) knots 0 0 0 0 1 1 1 1
  spline S980 degree 3 poles (-21.8571, 1.541) (-22.3737, 1.5626) (-22.8728, 1.5252) (-23.3816, 1.4341) knots 0 0 0 0 1 1 1 1
  spline S981 degree 3 poles (-23.3816, 1.4341) (-23.4094, 1.4293) (-23.4372, 1.4244) (-23.4658, 1.4193) knots 0 0 0 0 1 1 1 1
  spline S982 degree 3 poles (-23.4658, 1.4193) (-24.7424, 1.1917) (-24.7424, 1.1917) (-25.0402, 0.7675) knots 0 0 0 0 1 1 1 1
  spline S983 degree 3 poles (-25.0402, 0.7675) (-25.0535, 0.7413) (-25.0667, 0.715) (-25.0804, 0.688) knots 0 0 0 0 1 1 1 1
  spline S984 degree 3 poles (-25.0804, 0.688) (-25.1641, 0.535) (-25.2558, 0.435) (-25.3875, 0.3214) knots 0 0 0 0 1 1 1 1
  spline S985 degree 3 poles (-25.3875, 0.3214) (-25.4919, 0.3945) (-25.5183, 0.446) (-25.5787, 0.5562) knots 0 0 0 0 1 1 1 1
  spline S986 degree 3 poles (-25.5787, 0.5562) (-25.8637, 1.0186) (-26.322, 1.2384) (-26.7895, 1.4787) knots 0 0 0 0 1 1 1 1
  spline S987 degree 3 poles (-26.7895, 1.4787) (-26.8635, 1.5172) (-26.9374, 1.5558) (-27.0113, 1.5945) knots 0 0 0 0 1 1 1 1
  spline S988 degree 3 poles (-27.0113, 1.5945) (-27.043, 1.611) (-27.0746, 1.6275) (-27.1072, 1.6445) knots 0 0 0 0 1 1 1 1
  spline S989 degree 3 poles (-27.1072, 1.6445) (-27.2051, 1.6986) (-27.2979, 1.7583) (-27.3917, 1.8191) knots 0 0 0 0 1 1 1 1
  spline S990 degree 3 poles (-27.3917, 1.8191) (-27.8003, 2.0732) (-28.2527, 2.239) (-28.7065, 2.3931) knots 0 0 0 0 1 1 1 1
  spline S991 degree 3 poles (-28.7065, 2.3931) (-28.7426, 2.4055) (-28.7787, 2.4178) (-28.816, 2.4306) knots 0 0 0 0 1 1 1 1
  spline S992 degree 3 poles (-28.816, 2.4306) (-28.9039, 2.4607) (-28.9919, 2.4907) (-29.0799, 2.5206) knots 0 0 0 0 1 1 1 1
  spline S993 degree 3 poles (-29.0799, 2.5206) (-29.057, 2.5265) (-29.0341, 2.5324) (-29.0105, 2.5385) knots 0 0 0 0 1 1 1 1
  spline S994 degree 3 poles (-29.0105, 2.5385) (-28.7708, 2.6006) (-28.5312, 2.663) (-28.2916, 2.7256) knots 0 0 0 0 1 1 1 1
  spline S995 degree 3 poles (-28.2916, 2.7256) (-28.2024, 2.7489) (-28.1131, 2.7721) (-28.0238, 2.7952) knots 0 0 0 0 1 1 1 1
  spline S996 degree 3 poles (-28.0238, 2.7952) (-27.895, 2.8285) (-27.7662, 2.8622) (-27.6374, 2.8959) knots 0 0 0 0 1 1 1 1
  spline S997 degree 3 poles (-27.6374, 2.8959) (-27.5979, 2.9061) (-27.5585, 2.9162) (-27.5178, 2.9267) knots 0 0 0 0 1 1 1 1
  spline S998 degree 3 poles (-27.5178, 2.9267) (-26.8207, 3.1103) (-26.8207, 3.1103) (-26.6856, 3.3197) knots 0 0 0 0 1 1 1 1
  spline S999 degree 3 poles (-26.6856, 3.3197) (-26.4911, 3.7152) (-26.44, 4.1218) (-26.5265, 4.5551) knots 0 0 0 0 1 1 1 1
  spline S1000 degree 3 poles (-26.5265, 4.5551) (-26.6084, 4.7717) (-26.7872, 4.8764) (-26.9909, 4.9689) knots 0 0 0 0 1 1 1 1
  spline S1001 degree 3 poles (-26.9909, 4.9689) (-27.0923, 5.006) (-27.194, 5.0363) (-27.298, 5.0653) knots 0 0 0 0 1 1 1 1
  spline S1002 degree 3 poles (-27.298, 5.0653) (-27.3746, 5.0867) (-27.4512, 5.1081) (-27.5276, 5.13) knots 0 0 0 0 1 1 1 1
  spline S1003 degree 3 poles (-27.5276, 5.13) (-27.604, 5.1516) (-27.6806, 5.1725) (-27.7572, 5.1933) knots 0 0 0 0 1 1 1 1
  spline S1004 degree 3 poles (-27.7572, 5.1933) (-27.877, 5.2358) (-27.9544, 5.2726) (-28.0582, 5.3394) knots 0 0 0 0 1 1 1 1
  spline S1005 degree 3 poles (-28.0582, 5.3394) (-28.2637, 5.4661) (-28.4832, 5.5209) (-28.7157, 5.5795) knots 0 0 0 0 1 1 1 1
  spline S1006 degree 3 poles (-28.7157, 5.5795) (-28.7841, 5.5969) (-28.7841, 5.5969) (-28.8539, 5.6147) knots 0 0 0 0 1 1 1 1
  spline S1007 degree 3 poles (-28.8539, 5.6147) (-29.537, 5.7812) (-30.1909, 5.8267) (-30.8892, 5.7539) knots 0 0 0 0 1 1 1 1
  spline S1008 degree 3 poles (-30.8892, 5.7539) (-30.8832, 5.7785) (-30.8772, 5.803) (-30.871, 5.8283) knots 0 0 0 0 1 1 1 1
  spline S1009 degree 3 poles (-30.871, 5.8283) (-30.8774, 5.9212) (-30.8774, 5.9212) (-30.9608, 5.9967) knots 0 0 0 0 1 1 1 1
  spline S1010 degree 3 poles (-30.9608, 5.9967) (-31.0168, 6.0329) (-31.0168, 6.0329) (-31.074, 6.0699) knots 0 0 0 0 1 1 1 1
  spline S1011 degree 3 poles (-31.074, 6.0699) (-31.1129, 6.0955) (-31.1517, 6.1211) (-31.1918, 6.1475) knots 0 0 0 0 1 1 1 1
  spline S1012 degree 3 poles (-31.1918, 6.1475) (-31.228, 6.1709) (-31.2642, 6.1942) (-31.3015, 6.2182) knots 0 0 0 0 1 1 1 1
  spline S1013 degree 3 poles (-31.3015, 6.2182) (-31.3453, 6.2488) (-31.389, 6.2795) (-31.4341, 6.311) knots 0 0 0 0 1 1 1 1
  spline S1014 degree 3 poles (-31.4341, 6.311) (-31.4681, 6.3348) (-31.5021, 6.3587) (-31.5372, 6.3832) knots 0 0 0 0 1 1 1 1
  spline S1015 degree 3 poles (-31.5372, 6.3832) (-31.5647, 6.4041) (-31.5922, 6.4251) (-31.6205, 6.4466) knots 0 0 0 0 1 1 1 1
  spline S1016 degree 3 poles (-31.6205, 6.4466) (-31.7437, 6.5269) (-31.8658, 6.5762) (-32.0032, 6.6287) knots 0 0 0 0 1 1 1 1
  spline S1017 degree 3 poles (-32.0032, 6.6287) (-32.0297, 6.6389) (-32.0561, 6.6491) (-32.0834, 6.6596) knots 0 0 0 0 1 1 1 1
  spline S1018 degree 3 poles (-32.0834, 6.6596) (-32.1675, 6.692) (-32.2518, 6.7241) (-32.3361, 6.7561) knots 0 0 0 0 1 1 1 1
  spline S1019 degree 3 poles (-32.3361, 6.7561) (-32.4196, 6.7881) (-32.503, 6.8201) (-32.5865, 6.8522) knots 0 0 0 0 1 1 1 1
  spline S1020 degree 3 poles (-32.5865, 6.8522) (-32.6403, 6.8728) (-32.6941, 6.8933) (-32.7481, 6.9137) knots 0 0 0 0 1 1 1 1
  spline S1021 degree 3 poles (-32.7481, 6.9137) (-32.8913, 6.968) (-33.0309, 7.027) (-33.1703, 7.0907) knots 0 0 0 0 1 1 1 1
  spline S1022 degree 3 poles (-33.1703, 7.0907) (-33.3233, 7.1422) (-33.3233, 7.1422) (-33.4466, 7.1244) knots 0 0 0 0 1 1 1 1
  spline S1023 degree 3 poles (-33.4466, 7.1244) (-33.5848, 7.0433) (-33.6937, 6.9434) (-33.8052, 6.8301) knots 0 0 0 0 1 1 1 1
  spline S1024 degree 3 poles (-33.8052, 6.8301) (-34.0016, 6.6299) (-34.0016, 6.6299) (-34.2215, 6.4572) knots 0 0 0 0 1 1 1 1
  spline S1025 degree 3 poles (-34.2215, 6.4572) (-34.6995, 6.1043) (-34.7861, 5.5306) (-34.8812, 4.9674) knots 0 0 0 0 1 1 1 1
  spline S1026 degree 3 poles (-34.8812, 4.9674) (-34.8766, 4.941) (-34.8719, 4.9145) (-34.8671, 4.8873) knots 0 0 0 0 1 1 1 1
  spline S1027 degree 3 poles (-34.8671, 4.8873) (-34.8904, 4.8923) (-34.9138, 4.8974) (-34.9378, 4.9025) knots 0 0 0 0 1 1 1 1
  spline S1028 degree 3 poles (-34.9378, 4.9025) (-35.0465, 4.9259) (-35.1554, 4.9491) (-35.2642, 4.9722) knots 0 0 0 0 1 1 1 1
  spline S1029 degree 3 poles (-35.2642, 4.9722) (-35.3034, 4.9806) (-35.3427, 4.9891) (-35.3831, 4.9978) knots 0 0 0 0 1 1 1 1
  spline S1030 degree 3 poles (-35.3831, 4.9978) (-35.5919, 5.0419) (-35.7962, 5.0765) (-36.009, 5.0964) knots 0 0 0 0 1 1 1 1
  spline S1031 degree 3 poles (-36.009, 5.0964) (-36.3541, 5.1443) (-36.5652, 5.3677) (-36.7722, 5.6331) knots 0 0 0 0 1 1 1 1
  spline S1032 degree 3 poles (-36.7722, 5.6331) (-36.8641, 5.7647) (-36.9307, 5.8877) (-36.9713, 6.0446) knots 0 0 0 0 1 1 1 1
  spline S1033 degree 3 poles (-36.9713, 6.0446) (-36.93, 6.0682) (-36.93, 6.0682) (-36.8879, 6.0923) knots 0 0 0 0 1 1 1 1
  spline S1034 degree 3 poles (-36.8879, 6.0923) (-36.784, 6.1608) (-36.7137, 6.2296) (-36.6303, 6.3216) knots 0 0 0 0 1 1 1 1
  spline S1035 degree 3 poles (-36.6303, 6.3216) (-35.9723, 7.0157) (-35.2211, 7.6265) (-34.5007, 8.2547) knots 0 0 0 0 1 1 1 1
  spline S1036 degree 3 poles (-34.5007, 8.2547) (-33.785, 8.879) (-33.0973, 9.5191) (-32.4627, 10.2268) knots 0 0 0 0 1 1 1 1
  spline S1037 degree 3 poles (-32.4627, 10.2268) (-32.4451, 10.2088) (-32.4274, 10.1908) (-32.4092, 10.1722) knots 0 0 0 0 1 1 1 1
  spline S1038 degree 3 poles (-32.4092, 10.1722) (-32.0575, 9.8145) (-31.7032, 9.4616) (-31.3264, 9.1303) knots 0 0 0 0 1 1 1 1
  spline S1039 degree 3 poles (-31.3264, 9.1303) (-31.1837, 9.0046) (-31.0471, 8.8776) (-30.9171, 8.7388) knots 0 0 0 0 1 1 1 1
  spline S1040 degree 3 poles (-30.9171, 8.7388) (-30.5101, 8.3132) (-30.1527, 8.1968) (-29.574, 8.1338) knots 0 0 0 0 1 1 1 1
  spline S1041 degree 3 poles (-29.574, 8.1338) (-29.5084, 8.1252) (-29.4428, 8.1165) (-29.3772, 8.1077) knots 0 0 0 0 1 1 1 1
  spline S1042 degree 3 poles (-29.3772, 8.1077) (-28.6438, 8.0188) (-27.9174, 8.0735) (-27.1848, 8.142) knots 0 0 0 0 1 1 1 1
  spline S1043 degree 3 poles (-27.1848, 8.142) (-27.0333, 8.1561) (-26.8818, 8.17) (-26.7303, 8.1834) knots 0 0 0 0 1 1 1 1
  spline S1044 degree 3 poles (-26.7303, 8.1834) (-26.6934, 8.1868) (-26.6565, 8.1901) (-26.6185, 8.1935) knots 0 0 0 0 1 1 1 1
  spline S1045 degree 3 poles (-26.6185, 8.1935) (-26.3222, 8.2187) (-26.0268, 8.2275) (-25.7295, 8.224) knots 0 0 0 0 1 1 1 1
  spline S1046 degree 3 poles (-25.7295, 8.224) (-25.4397, 8.2252) (-25.2695, 8.3218) (-25.0565, 8.5173) knots 0 0 0 0 1 1 1 1
  spline S1047 degree 3 poles (-25.0565, 8.5173) (-24.9242, 8.5999) (-24.8512, 8.6377) (-24.6958, 8.6532) knots 0 0 0 0 1 1 1 1
  spline S1048 degree 3 poles (-24.6958, 8.6532) (-24.4841, 8.7055) (-24.3698, 8.8291) (-24.2316, 8.9932) knots 0 0 0 0 1 1 1 1
  spline S1049 degree 3 poles (-24.2316, 8.9932) (-24.1195, 9.1809) (-24.1288, 9.3727) (-24.1703, 9.5823) knots 0 0 0 0 1 1 1 1
  spline S1050 degree 3 poles (-24.1703, 9.5823) (-24.2817, 9.9169) (-24.5269, 10.198) (-24.7398, 10.4737) knots 0 0 0 0 1 1 1 1
  spline S1051 degree 3 poles (-24.7398, 10.4737) (-24.7778, 10.5239) (-24.8146, 10.5749) (-24.8506, 10.6265) knots 0 0 0 0 1 1 1 1
  spline S1052 degree 3 poles (-24.8506, 10.6265) (-25.0198, 10.8677) (-25.0198, 10.8677) (-25.1822, 10.9142) knots 0 0 0 0 1 1 1 1
  spline S1053 degree 3 poles (-25.1822, 10.9142) (-25.4781, 11.0159) (-25.7069, 11.2146) (-25.9398, 11.4183) knots 0 0 0 0 1 1 1 1
  spline S1054 degree 3 poles (-25.9398, 11.4183) (-25.5444, 11.2634) (-25.1618, 11.083) (-24.7776, 10.9027) knots 0 0 0 0 1 1 1 1
  spline S1055 degree 3 poles (-24.7776, 10.9027) (-24.4919, 10.7687) (-24.2046, 10.638) (-23.9172, 10.5075) knots 0 0 0 0 1 1 1 1
  spline S1056 degree 3 poles (-23.9172, 10.5075) (-23.8009, 10.4547) (-23.6847, 10.4016) (-23.5685, 10.3486) knots 0 0 0 0 1 1 1 1
  spline S1057 degree 3 poles (-23.5685, 10.3486) (-23.3419, 10.2452) (-23.1153, 10.142) (-22.8884, 10.0394) knots 0 0 0 0 1 1 1 1
  spline S1058 degree 3 poles (-22.8884, 10.0394) (-22.8505, 10.0223) (-22.8126, 10.0051) (-22.7735, 9.9874) knots 0 0 0 0 1 1 1 1
  spline S1059 degree 3 poles (-22.7735, 9.9874) (-22.7002, 9.9543) (-22.627, 9.9212) (-22.5537, 9.8881) knots 0 0 0 0 1 1 1 1
  spline S1060 degree 3 poles (-22.5537, 9.8881) (-22.503, 9.8652) (-22.503, 9.8652) (-22.4513, 9.8418) knots 0 0 0 0 1 1 1 1
  spline S1061 degree 3 poles (-22.4513, 9.8418) (-22.4218, 9.8285) (-22.3923, 9.8152) (-22.3619, 9.8015) knots 0 0 0 0 1 1 1 1
  spline S1062 degree 3 poles (-22.3619, 9.8015) (-22.3034, 9.7745) (-22.2453, 9.7467) (-22.1885, 9.7163) knots 0 0 0 0 1 1 1 1
  spline S1063 degree 3 poles (-22.1885, 9.7163) (-21.9936, 9.6149) (-21.8307, 9.5775) (-21.6123, 9.5674) knots 0 0 0 0 1 1 1 1
  spline S1064 degree 3 poles (-21.6123, 9.5674) (-21.5658, 9.5644) (-21.5658, 9.5644) (-21.5185, 9.5615) knots 0 0 0 0 1 1 1 1
  spline S1065 degree 3 poles (-21.5185, 9.5615) (-21.4183, 9.5554) (-21.3182, 9.5503) (-21.218, 9.5452) knots 0 0 0 0 1 1 1 1
  spline S1066 degree 3 poles (-21.218, 9.5452) (-21.1484, 9.5413) (-21.0788, 9.5374) (-21.0092, 9.5334) knots 0 0 0 0 1 1 1 1
  spline S1067 degree 3 poles (-21.0092, 9.5334) (-20.4466, 9.5024) (-19.8842, 9.482) (-19.3206, 9.4874) knots 0 0 0 0 1 1 1 1
  spline S1068 degree 3 poles (-19.3206, 9.4874) (-19.2891, 9.4876) (-19.2575, 9.4878) (-19.225, 9.488) knots 0 0 0 0 1 1 1 1
  spline S1069 degree 3 poles (-19.225, 9.488) (-18.1292, 9.5018) (-16.7384, 9.7508) (-15.913, 10.5426) knots 0 0 0 0 1 1 1 1
  spline S1070 degree 3 poles (-15.913, 10.5426) (-15.7382, 10.7656) (-15.6089, 11.0119) (-15.6224, 11.3025) knots 0 0 0 0 1 1 1 1
  spline S1071 degree 3 poles (-15.6224, 11.3025) (-15.6863, 11.7846) (-16.0023, 12.0234) (-16.3668, 12.3103) knots 0 0 0 0 1 1 1 1
  spline S1072 degree 3 poles (-16.3668, 12.3103) (-16.8909, 12.6992) (-17.4415, 12.8815) (-18.0684, 13.0434) knots 0 0 0 0 1 1 1 1
  spline S1073 degree 3 poles (-18.0684, 13.0434) (-18.3707, 13.1253) (-18.6252, 13.2381) (-18.8935, 13.3979) knots 0 0 0 0 1 1 1 1
  spline S1074 degree 3 poles (-18.8935, 13.3979) (-19.3521, 13.6695) (-19.8084, 13.7489) (-20.3289, 13.6199) knots 0 0 0 0 1 1 1 1
  spline S1075 degree 3 poles (-20.3289, 13.6199) (-20.5709, 13.5372) (-20.7719, 13.3642) (-20.9673, 13.2038) knots 0 0 0 0 1 1 1 1
  spline S1076 degree 3 poles (-20.9673, 13.2038) (-21.0003, 13.2287) (-21.0003, 13.2287) (-21.034, 13.2542) knots 0 0 0 0 1 1 1 1
  spline S1077 degree 3 poles (-21.034, 13.2542) (-21.681, 13.7272) (-22.4516, 13.9242) (-23.232, 14.051) knots 0 0 0 0 1 1 1 1
  spline S1078 degree 3 poles (-23.232, 14.051) (-23.9763, 14.1741) (-24.6236, 14.5053) (-25.27, 14.8822) knots 0 0 0 0 1 1 1 1
  spline S1079 degree 3 poles (-25.27, 14.8822) (-25.294, 14.896) (-25.3179, 14.9098) (-25.3425, 14.9239) knots 0 0 0 0 1 1 1 1
  spline S1080 degree 3 poles (-25.3425, 14.9239) (-25.9243, 15.2588) (-26.4859, 15.6239) (-27.0332, 16.0126) knots 0 0 0 0 1 1 1 1
  spline S1081 degree 3 poles (-27.0332, 16.0126) (-27.1228, 16.0743) (-27.2132, 16.1308) (-27.3071, 16.1857) knots 0 0 0 0 1 1 1 1
  spline S1082 degree 3 poles (-27.3071, 16.1857) (-27.4896, 16.2931) (-27.661, 16.4146) (-27.8337, 16.5369) knots 0 0 0 0 1 1 1 1
  spline S1083 degree 3 poles (-27.8337, 16.5369) (-28.0321, 16.6772) (-28.2298, 16.8138) (-28.4401, 16.9359) knots 0 0 0 0 1 1 1 1
  spline S1084 degree 3 poles (-28.4401, 16.9359) (-28.5356, 16.993) (-28.6281, 17.0538) (-28.7209, 17.1152) knots 0 0 0 0 1 1 1 1
  spline S1085 degree 3 poles (-28.7209, 17.1152) (-29.3537, 17.5298) (-30.124, 18.008) (-30.9074, 17.8632) knots 0 0 0 0 1 1 1 1
  spline S1086 degree 3 poles (-30.9074, 17.8632) (-31.0398, 17.8256) (-31.1407, 17.7437) (-31.2552, 17.6685) knots 0 0 0 0 1 1 1 1
  spline S1087 degree 3 poles (-31.2552, 17.6685) (-31.3254, 17.648) (-31.3962, 17.6296) (-31.4674, 17.613) knots 0 0 0 0 1 1 1 1
  spline S1088 degree 3 poles (-31.4674, 17.613) (-31.8172, 17.5249) (-32.0335, 17.3244) (-32.2801, 17.0698) knots 0 0 0 0 1 1 1 1
  spline S1089 degree 3 poles (-32.2801, 17.0698) (-32.3791, 16.9688) (-32.481, 16.8718) (-32.5848, 16.7757) knots 0 0 0 0 1 1 1 1
  spline S1090 degree 3 poles (-32.5848, 16.7757) (-32.617, 16.7458) (-32.6492, 16.7159) (-32.6824, 16.685) knots 0 0 0 0 1 1 1 1
  spline S1091 degree 3 poles (-32.6824, 16.685) (-32.7566, 16.6121) (-32.7566, 16.6121) (-32.8436, 16.6035) knots 0 0 0 0 1 1 1 1
  spline S1092 degree 3 poles (-32.8436, 16.6035) (-32.8609, 16.6312) (-32.8782, 16.6588) (-32.896, 16.6872) knots 0 0 0 0 1 1 1 1
  spline S1093 degree 3 poles (-32.896, 16.6872) (-33.2135, 17.1932) (-33.534, 17.6965) (-33.8742, 18.1877) knots 0 0 0 0 1 1 1 1
  spline S1094 degree 3 poles (-33.8742, 18.1877) (-33.8992, 18.2239) (-33.9241, 18.2601) (-33.9498, 18.2975) knots 0 0 0 0 1 1 1 1
  spline S1095 degree 3 poles (-33.9498, 18.2975) (-34.064, 18.4608) (-34.1797, 18.6215) (-34.3055, 18.7762) knots 0 0 0 0 1 1 1 1
  spline S1096 degree 3 poles (-34.3055, 18.7762) (-34.6205, 19.1647) (-34.8641, 19.5705) (-35.0993, 20.0112) knots 0 0 0 0 1 1 1 1
  spline S1097 degree 3 poles (-35.0993, 20.0112) (-35.5267, 20.8108) (-36.0105, 21.6081) (-36.9172, 21.9228) knots 0 0 0 0 1 1 1 1
  spline S1098 degree 3 poles (-36.9172, 21.9228) (-37.0913, 21.9594) (-37.2565, 21.9237) (-37.4289, 21.8904) knots 0 0 0 0 1 1 1 1
  spline S1099 degree 3 poles (-37.4289, 21.8904) (-37.4678, 21.8831) (-37.5066, 21.8758) (-37.5466, 21.8683) knots 0 0 0 0 1 1 1 1
  spline S1100 degree 3 poles (-37.5466, 21.8683) (-38.3823, 21.6952) (-38.9884, 21.1445) (-39.5214, 20.5068) knots 0 0 0 0 1 1 1 1
  spline S1101 degree 3 poles (-39.5214, 20.5068) (-39.5486, 20.4751) (-39.5758, 20.4434) (-39.6038, 20.4107) knots 0 0 0 0 1 1 1 1
  spline S1102 degree 3 poles (-39.6038, 20.4107) (-39.7638, 20.2192) (-39.8932, 20.0166) (-40.0164, 19.8) knots 0 0 0 0 1 1 1 1
  spline S1103 degree 3 poles (-40.0164, 19.8) (-40.0388, 19.7605) (-40.0612, 19.7211) (-40.0844, 19.6805) knots 0 0 0 0 1 1 1 1
  spline S1104 degree 3 poles (-40.0844, 19.6805) (-40.1778, 19.515) (-40.2706, 19.3492) (-40.3602, 19.1815) knots 0 0 0 0 1 1 1 1
  spline S1105 degree 3 poles (-40.3602, 19.1815) (-40.5125, 18.8967) (-40.6813, 18.6249) (-40.8569, 18.3542) knots 0 0 0 0 1 1 1 1
  spline S1106 degree 3 poles (-40.8569, 18.3542) (-40.923, 18.2523) (-40.9887, 18.1501) (-41.0544, 18.048) knots 0 0 0 0 1 1 1 1
  spline S1107 degree 3 poles (-41.0544, 18.048) (-41.0856, 17.9994) (-41.1169, 17.9508) (-41.1482, 17.9023) knots 0 0 0 0 1 1 1 1
  spline S1108 degree 3 poles (-41.1482, 17.9023) (-41.179, 17.8545) (-41.2097, 17.8066) (-41.2402, 17.7586) knots 0 0 0 0 1 1 1 1
  spline S1109 degree 3 poles (-41.2402, 17.7586) (-41.2802, 17.6959) (-41.3208, 17.6336) (-41.3616, 17.5714) knots 0 0 0 0 1 1 1 1
  spline S1110 degree 3 poles (-41.3616, 17.5714) (-41.5465, 17.2846) (-41.6929, 16.9906) (-41.8309, 16.6789) knots 0 0 0 0 1 1 1 1
  spline S1111 degree 3 poles (-41.8309, 16.6789) (-42.0704, 16.1135) (-42.0704, 16.1135) (-42.5077, 15.6951) knots 0 0 0 0 1 1 1 1
  spline S1112 degree 3 poles (-42.5077, 15.6951) (-42.6276, 15.6587) (-42.7094, 15.6838) (-42.8309, 15.7125) knots 0 0 0 0 1 1 1 1
  spline S1113 degree 3 poles (-42.8309, 15.7125) (-42.8779, 15.7234) (-42.9248, 15.7343) (-42.9731, 15.7456) knots 0 0 0 0 1 1 1 1
  spline S1114 degree 3 poles (-42.9731, 15.7456) (-43.0476, 15.7637) (-43.0476, 15.7637) (-43.1237, 15.7823) knots 0 0 0 0 1 1 1 1
  spline S1115 degree 3 poles (-43.1237, 15.7823) (-43.1743, 15.7942) (-43.2249, 15.8061) (-43.277, 15.8184) knots 0 0 0 0 1 1 1 1
  spline S1116 degree 3 poles (-43.277, 15.8184) (-43.5852, 15.892) (-43.888, 15.9728) (-44.1875, 16.0763) knots 0 0 0 0 1 1 1 1
  spline S1117 degree 3 poles (-44.1875, 16.0763) (-44.3054, 16.104) (-44.3939, 16.111) (-44.5135, 16.111) knots 0 0 0 0 1 1 1 1
  spline S1118 degree 3 poles (-44.5135, 16.111) (-44.7686, 16.1124) (-45.0072, 16.166) (-45.2558, 16.2195) knots 0 0 0 0 1 1 1 1
  spline S1119 degree 3 poles (-45.2558, 16.2195) (-46.3261, 16.4374) (-47.3716, 16.5413) (-48.4437, 16.2899) knots 0 0 0 0 1 1 1 1
  spline S1120 degree 3 poles (-48.4437, 16.2899) (-48.4742, 16.2832) (-48.5047, 16.2765) (-48.5362, 16.2696) knots 0 0 0 0 1 1 1 1
  spline S1121 degree 3 poles (-48.5362, 16.2696) (-49.2063, 16.1143) (-49.7697, 15.7409) (-50.344, 15.3773) knots 0 0 0 0 1 1 1 1